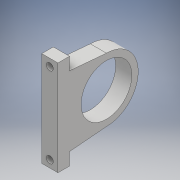
# Autodesk Inventor part: mount
Saved by Autodesk Inventor 2017 (Build 210142000, 142)
## iProperties
Created: 2017-04-28
Part Number: mount
Material: Generic
Document SubType Name: Modeling
Designer: s4321966
Density: 1 g/cm^3
Appearance: Default
Author: s4321966
Autodesk Inventor part; units mm, degrees
ref_plane "YZ Plane" through (0, 0, 0) normal (1, 0, 0) x (0, 1, 0)
ref_plane "XZ Plane" through (0, 0, 0) normal (0, 1, 0) x (-1, 0, 0)
ref_plane "XY Plane" through (0, 0, 0) normal (0, 0, 1) x (1, 0, 0)
sketch "Sketch1" plane through (0, 0, 0) normal (1, 0, 0) x (0, 1, 0)
  circle A0 centre (0, 0) radius 11
  line L0 (0, 0) -> (0, -21)
  line L1 (0, 0) -> (21, 0) construction
  line L2 (0, 0) -> (-21, 0)
  line L3 (0, 0) -> (21, 0) construction
  circle A1 centre (0, 0) radius 13.75
  line L4 (0, -13.75) -> (28.06, -13.75) construction
  line L5 (-21, 0) -> (-21, -15.5873)
  line L6 (-21, -15.5873) -> (0, -13.75)
  line L7 (-21, 0) -> (-21, 15.5873)
  line L8 (-21, 15.5873) -> (0, 13.75)
  line L9 (-21, 15.5873) -> (-21, 20.5873)
  line L10 (-21, 15.5873) -> (-16, 15.5873) construction
  line L11 (-21, 20.5873) -> (-16, 20.5873)
  line L12 (-16, 20.5873) -> (-21, 20.5873)
  line L13 (-21, 20.5873) -> (-21, 0)
  line L14 (-21, 0) -> (-16, 0)
  line L15 (-16, 0) -> (-16, 20.5873)
  line L16 (-21, 0) -> (-21, -15.5873)
  line L17 (-21, -15.5873) -> (-21, -20.5873)
  line L18 (-21, -15.5873) -> (-16, -15.5873) construction
  line L19 (-21, -20.5873) -> (-16, -20.5873)
  line L20 (-16, -20.5873) -> (-21, -20.5873)
  line L21 (-21, -20.5873) -> (-21, 0)
  line L22 (-16, 0) -> (-16, -20.5873)
  line L23 (0, 13.75) -> (-8.1531, 9.4095)
  line L24 (-8.1531, 9.4095) -> (-12.797, 1.5106)
  line L25 (-12.797, 1.5106) -> (-11.2995, -5.5298)
  line L26 (-11.2995, -5.5298) -> (-6.7209, -9.817)
  line L27 (-6.7209, -9.817) -> (0, -13.75)
  line L28 (-16, 15.1498) -> (-16, -15.1498)
  dimension "d6" = 27.5
  dimension "d0" = 22
  dimension "d1" = 21
  dimension "d2" = 90
  dimension "d3" = 21
  dimension "d4" = 180
  dimension "d8" = 5
  dimension "d9" = 90
  dimension "d10" = 5
  dimension "d11" = 90
  constraints: 58 end point, 6 horizontal, 6 symmetric about line, 5 point on line, 3 equal length, 3 vertical, 2 parallel, 2 perpendicular, 1 centre point, 1 coincident, 1 vertical alignment, 2 other
  measures "d0" diameter of A0
  measures "d1" distance of L0.start L0.end
  measures "d2" angle of L0 L1
  measures "d3" distance of L0.start L2.end
  measures "d4" angle of L2 L3
  measures "d8" distance of L7.end L9.end
  measures "d9" angle of L10 L9
  measures "d10" distance of L9.end L11.end
  measures "d11" angle of L9 L11
extrude "Extrusion1" add sketch "Sketch1" along normal blind 7 contours A0 L2 L25 L24 L23 A1 L0 | A0 L0 L27 L26 L25 L2 | L25 L26 L27 A1 L2 | L2 A1 L23 L24 L25 | L6 L22 L2 A1 | L2 L15 L8 A1 | L22 L19 L17 L6 | L6 L5 L2 L22 | L2 L7 L8 L15 | L8 L9 L11 L15
sketch "Sketch2" plane through (0, -16, -15.1498) normal (0, 1, 0) x (1, 0, 0)
  line L0 (0, -35.7371) -> (0, 5.4374) projected
  line L1 (0, -15.1498) -> (0, 5.4374)
  line L2 (0, -15.1498) -> (23.9125, -15.1498)
  line L3 (7, -35.7371) -> (7, 5.4374) projected
  line L4 (7, -0.2045) -> (0, 4.7429)
  circle A0 centre (3.5, 2.2692) radius 1.5
  line L5 (7, -30.0951) -> (0, -35.0426)
  circle A1 centre (3.5, -32.5688) radius 1.5
  dimension "d14" = 3
  constraints: 8 end point, 3 symmetric about line, 2 centre point, 2 point on line, 1 collinear, 1 horizontal, 1 other
  measures "d14" diameter of A0
extrude "Extrusion2" cut sketch "Sketch2" against normal blind 7 contours A1 L5 | L5 A1 | A0 L4 | L4 A0
body "Solid1"
